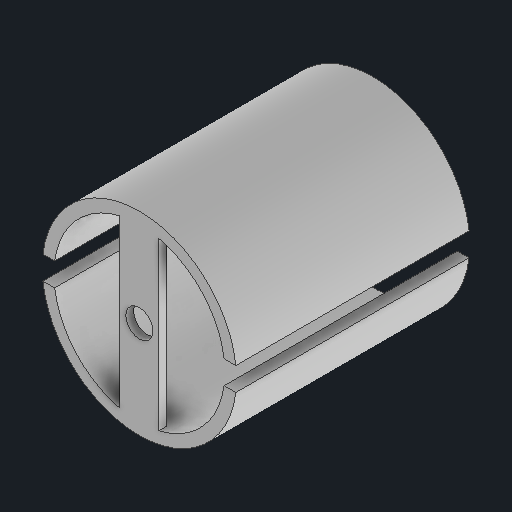
# Autodesk Inventor part: CatcherModel
Saved by Autodesk Inventor 2027 (Build 310192060, 192F)
## iProperties
Created: 2025-10-14
Part Number: CatcherModel
Material: Generisch
Document SubType Name: Modeling
Designer: Halle20
Density: 1 g/cm^3
Appearance: Vorgabe
Author: Halle20
Autodesk Inventor part; units mm, degrees
ref_plane "YZ Plane" through (0, 0, 0) normal (1, 0, 0) x (0, 1, 0)
ref_plane "XZ Plane" through (0, 0, 0) normal (0, 1, 0) x (-1, 0, 0)
ref_plane "XY Plane" through (0, 0, 0) normal (0, 0, 1) x (1, 0, 0)
sketch "Skizze1" plane through (0, 0, 0) normal (0, 1, 0) x (-1, 0, 0)
  circle A0 centre (0, 0) radius 12.5
  circle A1 centre (0, 0) radius 11
  dimension "d0" = 25
  dimension "d1" = 22
  constraints: 2 centre point, 2 coincident
  measures "d0" diameter of A0
  measures "d1" diameter of A1
extrude "Extrusion1" add sketch "Skizze1" along normal blind 30
sketch "Skizze2" plane through (0, 0, 0) normal (0, -1, 0) x (1, 0, 0)
  circle A0 centre (0, 0) radius 1.75
  line L0 (0, 0) -> (0, 3.5)
  line L1 (0, 3.5) -> (2.5, 3.5)
  line L2 (2.5, 3.5) -> (-2.5, 3.5)
  line L3 (-2.5, 3.5) -> (-2.5, -11.5)
  line L4 (-2.5, -11.5) -> (2.5, -11.5)
  line L5 (2.5, -11.5) -> (2.5, 3.5)
  line L6 (2.5, 3.5) -> (-2.5, 3.5)
  line L7 (-2.5, 3.5) -> (-2.5, 11.3675)
  line L8 (-2.5, 11.3675) -> (2.5, 11.3675)
  line L9 (2.5, 11.3675) -> (2.5, 3.5)
  dimension "d7" = 3.5
  dimension "d8" = 3.5
  dimension "d9" = 2.5
  dimension "d10" = 5
  dimension "d11" = 15
  constraints: 20 end point, 4 parallel, 3 perpendicular, 2 horizontal, 1 centre point, 1 coincident, 1 vertical
  measures "d7" diameter of A0
  measures "d8" distance of L0.start L0.end
  measures "d9" distance of L0.end L1.end
  measures "d10" distance of L4.end L3.end
  measures "d11" distance of L3.end L2.end
extrude "Extrusion2" add sketch "Skizze2" against normal blind 1
sketch "Skizze3" plane through (0, 30, 0) normal (0, 1, 0) x (1, 0, 0)
  line L0 (-17.8957, 0) -> (-17.8957, -1.5)
  line L1 (-17.8957, -1.5) -> (13.7177, -1.5)
  line L2 (13.7177, -1.5) -> (13.7177, 1.5)
  line L3 (13.7177, 1.5) -> (-17.8957, 1.5)
  line L4 (-17.8957, 1.5) -> (-17.8957, -1.5)
  point P0 (0, 0)
  dimension "d14" = 1.5
  dimension "d15" = 3
  constraints: 10 end point, 2 parallel, 1 horizontal, 1 perpendicular, 1 vertical
  measures "d14" distance of L0.start L0.end
  measures "d15" distance of L2.end L1.end
extrude "Extrusion3" cut sketch "Skizze3" against normal up to surface (29 mm away)
sketch "Skizze4" plane through (-12.4097, 1, -1.5) normal (0, 1, 0) x (1, 0, 0)
  line L0 (0, 0) -> (1.5124, 0) projected
  line L1 (0, 0) -> (-0.8042, 0)
  line L2 (-0.8042, 0) -> (2.2509, 0)
  line L3 (2.2509, 0) -> (2.2509, -3)
  line L4 (2.2509, -3) -> (-0.8042, -3)
  line L5 (-0.8042, -3) -> (-0.8042, 0)
  point P0 (12.4097, -1.5)
  dimension "d18" = 3
  constraints: 10 end point, 2 horizontal, 2 parallel, 1 perpendicular
  measures "d18" distance of L2.end L3.end
extrude "Extrusion4" cut sketch "Skizze4" against normal through all
sketch "Skizze5" plane through (10.8972, 1, 1.5) normal (0, 1, 0) x (1, 0, 0)
  line L0 (0, 0) -> (1.5124, 0) projected
  line L1 (0, 0) -> (2.0703, 0)
  line L2 (2.0703, 0) -> (2.0703, 3)
  line L3 (2.0703, 3) -> (0, 3)
  line L4 (0, 3) -> (0, 0)
  point P0 (-10.8972, 1.5)
  dimension "d24" = 3
  constraints: 8 end point, 2 parallel, 1 horizontal, 1 perpendicular
  measures "d24" distance of L2.end L1.end
extrude "Extrusion5" cut sketch "Skizze5" against normal blind 10
